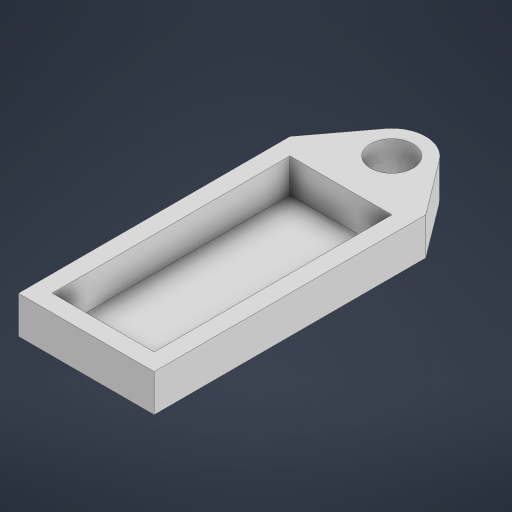
# Autodesk Inventor part: Bauteil1
Saved by Autodesk Inventor 2024.3 (Build 283343010, 343A)
## iProperties
Created: 2025-05-12
Part Number: Bauteil1
Material: Generisch
Document SubType Name: Modeling
Designer: David
Density: 1 g/cm^3
Appearance: Vorgabe
Author: David
## iProperties of the stored document Bauteil1_3D-Druck.ipt
Created: 2025-05-12
Part Number: Bauteil1_3D-Druck
Material: Generisch
Document SubType Name: Modeling
Designer: David
Density: 1 g/cm^3
Appearance: Vorgabe
Author: David
Autodesk Inventor part; units mm, degrees
ref_plane "YZ Plane" through (0, 0, 0) normal (1, 0, 0) x (0, 1, 0)
ref_plane "XZ Plane" through (0, 0, 0) normal (0, 1, 0) x (-1, 0, 0)
ref_plane "XY Plane" through (0, 0, 0) normal (0, 0, 1) x (1, 0, 0)
sketch "Skizze1" plane through (0, 0, 0) normal (0, 0, 1) x (1, 0, 0)
  circle A0 centre (0, 0) radius 6.25
  line L0 (-20, -90) -> (-20, -10)
  line L1 (-20, -10) -> (-8, 6)
  arc A1 (8, 6) -> (-8, 6) centre (0, 0) ccw
  line L2 (8, 6) -> (20, -10)
  line L3 (20, -10) -> (20, -90)
  line L4 (20, -90) -> (-20, -90)
  line L5 (-15, -15) -> (15, -15)
  line L6 (15, -15) -> (15, -85)
  line L7 (15, -85) -> (-15, -85)
  line L8 (-15, -85) -> (-15, -15)
  point P0 (0, -90)
  point P1 (0, -15)
  dimension "d0" = 12.5
  dimension "d1" = 30
  dimension "d2" = 70
  dimension "d3" = 15
  dimension "d4" = 5
  dimension "d5" = 5
  dimension "d6" = 5
  dimension "d7" = 10
  constraints: 18 end point, 3 parallel, 2 centre point, 2 coincident, 2 midpoint, 2 perpendicular, 2 point on circle, 2 tangent, 2 vertical alignment, 1 horizontal, 1 horizontal alignment, 1 vertical
  measures "d0" diameter of A0
  measures "d1" distance of L6.end L7.end
  measures "d2" distance of L5.end L6.end
  measures "d3" distance from line of point (0, 0) L5
  measures "d4" distance between parallel lines of L3 L6
  measures "d5" distance between parallel lines of L4 L7
  measures "d6" distance from line of L5 L2.end
  measures "d7" radius of A1
extrude "Extrusion1" add sketch "Skizze1" along normal blind 10
extrude "Extrusion2" add sketch "Skizze1" against normal blind 1 contours L0 L1 A1 L2 L3 L4 | L5 L6 L7 L8
